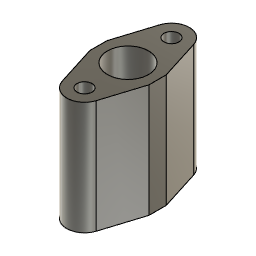
propeen corbuader v1 (Autodesk Fusion 360 design; units mm, degrees)
Autodesk Fusion 360 part; units mm, degrees
sketch "Sketch1" plane through (0, 0, 0) normal (0, 0, 1) x (1, 0, 0)
  circle A0 centre (0, 35) radius 3.65
  line L0 (0, 31.35) -> (0, 23.85)
  circle A1 centre (0, 13.85) radius 10
  line L1 (0, 23.85) -> (0, 3.85)
  line L2 (0, 3.85) -> (0, -3.65)
  circle A2 centre (0, -7.3) radius 3.65
  circle A3 centre (0, -7.3) radius 8.65
  circle A4 centre (0, 35) radius 8.65
  circle A5 centre (0, 13.85) radius 15
  line L3 (-14.4076, 18.0238) -> (-8.2514, 37.5955)
  line L4 (-14.4076, 18.0238) -> (14.4076, 18.0238)
  line L5 (-14.4076, 18.0238) -> (-14.4076, 9.6762)
  line L6 (-14.4076, 9.6762) -> (14.4076, 9.6762)
  line L7 (14.4076, 18.0238) -> (14.4076, 9.6762)
  line L8 (14.4076, 18.0238) -> (8.2514, 37.5955)
  line L9 (14.4076, 9.6762) -> (8.2514, -9.8955)
  line L10 (-14.4076, 9.6762) -> (-8.2514, -9.8955)
  dimension "d1" = 7.3
  dimension "d2" = 7.5
  dimension "d3" = 20
  dimension "d4" = 7.5
  dimension "d5" = 7.3
  dimension "d6" = 17.3
  dimension "d7" = 17.3
  dimension "d8" = 30
  constraint coincident A0 L0.start
  constraint vertical L0
  constraint coincident L0.end A1
  constraint coincident A1 L1.end
  constraint parallel L0 L1
  constraint parallel L1 L2
  constraint coincident L2.end A2
  constraint concentric A2 A3
  constraint concentric A0 A4
  constraint concentric A1 A5
  constraint coincident A5 L3.start
  constraint coincident A4 L3.end
  constraint tangent A4 L3
  constraint coincident A5 L4.end
  constraint horizontal L4
  constraint coincident A5 L5.end
  constraint perpendicular L4 L5
  constraint coincident A5 L6.end
  constraint perpendicular L5 L6
  constraint coincident A4 L8.end
  constraint tangent A4 L8
  constraint coincident A3 L9.end
  constraint tangent A3 L9
  constraint coincident A3 L10.end
  constraint tangent A3 L10
  constraint parallel L8 L10
  measures "d1" diameter of A0
  measures "d2" distance of L0.start L0.end
  measures "d3" diameter of A1
  measures "d4" distance of L1.end L2.end
  measures "d5" diameter of A2
  measures "d6" diameter of A3
  measures "d7" diameter of A4
  measures "d8" diameter of A5
extrude "Extrude1" add sketch "Sketch1" along normal blind 55 contours L0 A4 A5 | A4 A5 | L0 A4 A5 | L0 A1 A4 A5 L4 L8 | L0 A1 A4 A5 L3 L4 | A4 A5 L8 | A4 A5 L3 | A1 L4 L6 L7 | A1 L4 L5 L6 | A1 L2 A3 A5 L6 L10 | A1 L2 A3 A5 L6 L9 | A3 A5 L9 | A3 A5 L10 | L2 A3 A5 | L2 A3 A5 | A3 A5
